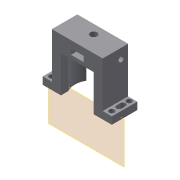
# Autodesk Inventor part: opentrons_Gearbox
Saved by Autodesk Inventor 2019.4 (Build 234330000, 330)
## iProperties
Created: 2021-01-24
Part Number: opentrons_Gearbox
Material: Generic
Document SubType Name: Modeling
Designer: diederichbenedict
Density: 1 g/cm^3
Appearance: Default
Author: diederichbenedict
Autodesk Inventor part; units mm, degrees
ref_plane "YZ Plane" through (0, 0, 0) normal (1, 0, 0) x (0, 1, 0)
ref_plane "XZ Plane" through (0, 0, 0) normal (0, 1, 0) x (-1, 0, 0)
ref_plane "XY Plane" through (0, 0, 0) normal (0, 0, 1) x (1, 0, 0)
ref_plane "Work Plane1" through (0, 0, 0) normal (0, 0, 1) x (1, 0, 0)
sketch "Sketch1" plane through (0, 0, 0) normal (0, 0, 1) x (1, 0, 0)
  line L0 (0, 0) -> (0, 20.9) projected
  line L1 (0, 0) -> (38, 0) projected
  line L2 (38, 0) -> (38, 20.9) projected
  line L3 (0, 20.9) -> (38, 20.9) projected
  line L4 (36.95, 20.9) -> (36.95, 0)
  line L5 (34.05, 20.9) -> (34.05, 0)
  line L6 (3.95, 20.9) -> (3.95, 0)
  line L7 (1.05, 20.9) -> (1.05, 0)
  line L8 (21, 26.7276) -> (21, 46.0982)
  line L9 (17, 26.7276) -> (17, 46.0982)
  line L10 (36.95, 20.9) -> (27.95, 20.9)
  line L11 (27.95, 20.9) -> (27.95, 24.9)
  line L12 (27.95, 24.9) -> (36.95, 24.9)
  line L13 (36.95, 24.9) -> (36.95, 20.9)
  line L14 (27.95, 24.9) -> (32.95, 24.9)
  line L15 (32.95, 24.9) -> (32.95, 49.9)
  line L16 (32.95, 49.9) -> (27.95, 49.9)
  line L17 (27.95, 49.9) -> (27.95, 24.9)
  line L18 (27.95, 49.9) -> (19, 49.9)
  line L19 (19, 40.95) -> (27.95, 40.95)
  line L20 (27.95, 40.95) -> (27.95, 49.9)
  line L21 (22.45, 42.95) -> (22.45, 45.9)
  line L22 (15.55, 45.9) -> (15.55, 42.95)
  line L23 (15.55, 42.95) -> (22.45, 45.9) construction
  line L24 (22.45, 42.95) -> (15.55, 45.9) construction
  line L25 (19, 49.9) -> (19, 45.9)
  line L26 (19, 42.95) -> (19, 40.95)
  line L27 (19, 46.0982) -> (19, 45.9)
  line L28 (19, 42.95) -> (19, 2.6115)
  line L29 (22.45, 45.9) -> (19, 45.9)
  line L30 (17, 45.9) -> (15.55, 45.9)
  line L31 (15.55, 42.95) -> (17, 42.95)
  line L32 (19, 42.95) -> (22.45, 42.95)
  line L33 (36.95, 24.9) -> (38, 24.9)
  line L34 (38, 24.9) -> (38, 20.9)
  line L35 (38, 20.9) -> (36.95, 20.9)
  line L36 (36.95, 20.9) -> (36.95, 24.9)
  dimension "d0" = 9
  dimension "d1" = 4
  dimension "d2" = 5
  dimension "d3" = 25
  dimension "d7" = 6.9
  dimension "d8" = 2.95
  dimension "d20" = 4
  dimension "d21" = 2
  constraints: 66 end point, 14 parallel, 8 vertical, 7 perpendicular, 6 horizontal, 3 point on line, 12 other
  measures "d0" distance of L11.end L12.end
  measures "d1" distance of L10.end L11.end
  measures "d2" distance of L16.end L15.end
  measures "d3" distance of L15.end L14.end
  measures "d7" distance of L22.start L21.end
  measures "d8" distance of L21.end L21.start
  measures "d20" distance between parallel lines of L29 L18
  measures "d21" distance between parallel lines of L19 L32
extrude "Extrusion1" add sketch "Sketch1" along normal blind 5 and the other way blind 9 contours L3 L11 L12 L13 | L26 L32 L8 L19 | L13 L33 L34 L3 | L17 L16 L15 L12 | L8 L32 L21 L29 L25 L18 L17 L19
sketch "Sketch2" plane through (19, 49.9, -9) normal (0, 1, 0) x (-1, 0, 0)
  circle A0 centre (0, 5) radius 2.2 projected
  circle A1 centre (0, 5) radius 1.9
  point P0 (19, 9)
  dimension "d19" = 3.8
  constraints: 1 centre point, 1 coincident
  measures "d19" diameter of A1
extrude "Extrusion2" cut sketch "Sketch2" against normal through all contours A1
sketch "Sketch3" plane through (32.95, 24.9, -9) normal (1, 0, 0) x (0, 0, 1)
  line L0 (5.7, 1.8276) -> (5.7, 21.1982)
  line L1 (1.7, 1.8276) -> (1.7, 21.1982)
  line L2 (0, -21) -> (14, -21) projected
  line L3 (0, -25) -> (0, 0) projected
  line L4 (0, 0) -> (14, 0) projected
  line L5 (14, 0) -> (14, -25) projected
  line L6 (14, -25) -> (0, -25) projected
  line L7 (0, -18.05) -> (14, -18.05) projected
  circle A0 centre (3.7717, -19.5574) radius 1.45
  point P0 (9, 24.9)
  dimension "d14" = 2.9
  constraints: 4 end point, 2 vertical, 1 centre point, 4 other
  measures "d14" diameter of A0
extrude "Extrusion3" cut sketch "Sketch3" against normal through all contours A0 L2 | L2 A0
sketch "Sketch4" plane through (27.95, 20.9, -9) normal (0, -1, 0) x (-1, 0, 0)
  circle A0 centre (8.95, -5) radius 3.1 projected
  circle A1 centre (8.95, -5) radius 10.2555
  circle A2 centre (-7.525, -11.5) radius 1.45 projected
  circle A3 centre (-7.55, -6.5) radius 1.45 projected
  circle A4 centre (-7.55, -2) radius 1.45 projected
  line L0 (-7.55, -7.5947) -> (-7.55, -5.4053) construction
  line L1 (-9, -7.5947) -> (-9, -5.4053)
  line L2 (-6.1, -5.4053) -> (-6.1, -7.5947)
  arc A5 (-9, -7.5947) -> (-6.1, -7.5947) centre (-7.55, -7.5947) ccw
  arc A6 (-6.1, -5.4053) -> (-9, -5.4053) centre (-7.55, -5.4053) ccw
  point P0 (27.95, -9)
  constraints: 8 end point, 4 point on circle, 4 tangent, 3 centre point, 1 coincident, 1 midpoint, 1 parallel, 1 vertical
extrude "Extrusion4" cut sketch "Sketch4" against normal up to surface (20.05 mm away) contours A0 | A1 | A2 | A3 | L2 A5 L1 A3 | A3 L1 A6 L2 | A4
mirror "Mirror1" about plane through (19, 49.9, 0) normal (-1, 0, 0) of "Extrusion1", "Extrusion2", "Extrusion3", "Extrusion4"
body "Solid1"
